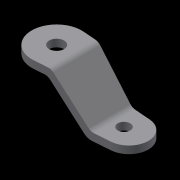
# Autodesk Inventor part: ShoulderConnectorBodyFinal
Saved by Autodesk Inventor 2015 (Build 190159000, 159)
## iProperties
Created: 2014-09-27
Part Number: ShoulderConnectorBodyFinal
Material: Generic
Document SubType Name: Modeling
Designer: Inventor
Density: 1 g/cm^3
Appearance: Default
Mass: 7.33645 g
Surface Area: 44.888 cm^2
Volume: 7.33645 cm^3
RuleStatus: InUse
CX: 52.70 mm
CY: 30.70 mm
CZ: 18.00 mm
Author: Inventor
Autodesk Inventor part; units mm, degrees
ref_plane "YZ Plane" through (0, 0, 0) normal (1, 0, 0) x (0, 1, 0)
sketch "Body" plane through (0, 0, 0) normal (0, 0, 1) x (1, 0, 0)
  circle A0 centre (0, 0) radius 10
  line L0 (0, 0) -> (29, 0) construction
  circle A1 centre (29, 0) radius 7.75
  line L1 (0.7759, 9.9699) -> (29.6013, 7.7266)
  line L2 (0.7759, -9.9699) -> (29.6013, -7.7266)
  dimension "SmallDiameter" = 20
  dimension "d1" = 29
  dimension "LargeDiameter" = 15.5
  constraints: 6 end point, 4 point on circle, 4 tangent, 2 centre point, 2 coincident, 1 horizontal
  measures "SmallDiameter" diameter of A0
  measures "d1" distance of L0.start L0.end
  measures "LargeDiameter" diameter of A1
extrude "BodyFeature" add sketch "Body" along normal blind 18
ref_plane "SideProfilePlane" through (0, 12, 0) normal (0, 1, 0) x (-1, 0, 0)
sketch "SideProfile" plane through (0, 12, 0) normal (0, 1, 0) x (-1, 0, 0)
  line L0 (10, 18) -> (-0.7759, 18) construction
  line L1 (10, 18) -> (10, 15)
  line L2 (10, 15) -> (-6, 15)
  line L3 (-6, 15) -> (-20.75, 0)
  line L4 (-20.75, 0) -> (-36.75, 0)
  line L5 (-29.6013, 0) -> (-0.7759, 0) construction
  line L6 (-36.75, 0) -> (-36.75, 18) construction
  line L7 (-29.6013, 18) -> (-36.75, 18) construction
  line L8 (-29.6013, 18) -> (-0.7759, 18) construction
  line L9 (-22.0074, 3) -> (-7.2574, 18)
  line L10 (-36.75, 3) -> (-22.0074, 3)
  line L11 (-36.75, 0) -> (-36.75, 3)
  line L12 (10, 18) -> (-7.2574, 18)
  dimension "Thickness" = 3
  dimension "d15" = 3
  dimension "d16" = 3
  dimension "d17" = 16
  dimension "d18" = 16
  constraints: 16 end point, 4 collinear, 1 horizontal, 1 parallel, 1 vertical
  measures "Thickness" distance of L0.start L1.end
  measures "d15" distance between parallel lines of L3 L9
  measures "d16" distance of L10.start L4.end
  measures "d17" distance of L1.end L2.end
  measures "d18" distance of L3.end L4.end
extrude "SideProfileFeature" cut sketch "SideProfile" against normal through all keep common part
fillet "BodyFilletsFeate" radius 3 3 edges at (6, 0, 15) (22.0074, 0, 3) (7.2574, 0, 18)
ref_plane "HeadMountPlane" through (29, 0, 3) normal (0, 0, 1) x (1, 0, 0)
sketch "HeadMountHole" plane through (29, 0, 3) normal (0, 0, 1) x (1, 0, 0)
  circle A0 centre (-2, 0) radius 3.25
  arc A1 (0.6013, -7.7266) -> (0.6013, 7.7266) centre (0, 0) ccw construction
  line L0 (-2, 0) -> (0, 0) construction
  point P0 (-29, 0)
  dimension "d307" = 2
  dimension "d308" = 6.5
  constraints: 2 end point, 1 centre point, 1 horizontal
  measures "d307" distance of L0.end L0.start
  measures "d308" diameter of A0
hole "HeadMountHoleFeature" at (27, 0, 3) direction (0, 0, -1) diameter 5 end through all
sketch "BodyMountHole" plane through (0, 0, 18) normal (0, 0, 1) x (1, 0, 0)
  arc A0 (0.7759, 9.9699) -> (0.7759, -9.9699) centre (0, 0) ccw projected
hole "BodyMountHoleFeature" at (0, 0, 18) direction (0, 0, -1) diameter 6 end through all
fillet "BodyFillets2Feature" radius 4 1 edges at (20.75, 0, 0)
equation "\"d16\" = Thickness"
